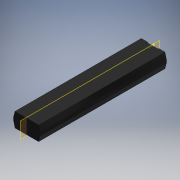
# Autodesk Inventor part: atmega_mold
Saved by Autodesk Inventor 2018 (Build 220112000, 112)
## iProperties
Created: 2017-04-13
Part Number: atmega_mold
Material: Generic
Document SubType Name: Modeling
Designer: kampe_000
Density: 1 g/cm^3
Appearance: Default
atmegaPinDistance: 2,540 mm
AtmegaChamfer_D2: 1,500 mm
AtmegaChamfer_D1: 0,400 mm
Author: kampe_000
Autodesk Inventor part; units mm, degrees
ref_plane "YZ Plane" through (0, 0, 0) normal (1, 0, 0) x (0, 1, 0)
ref_plane "XZ Plane" through (0, 0, 0) normal (0, 1, 0) x (-1, 0, 0)
ref_plane "XY Plane" through (0, 0, 0) normal (0, 0, 1) x (1, 0, 0)
sketch "Sketch1" plane through (0, 0, 0) normal (0, 1, 0) x (-1, 0, 0)
  line L0 (0, 0) -> (7.3, 0)
  line L1 (7.3, 0) -> (7.3, -34.6)
  line L2 (7.3, -34.6) -> (0, -34.6)
  line L3 (0, -34.6) -> (0, 0)
  dimension "d0" = 7.3
  dimension "d1" = 34.6
  constraints: 8 end point, 2 parallel, 1 horizontal, 1 perpendicular
  measures "d0" distance of L1.end L2.end
  measures "d1" distance of L0.end L1.end
extrude "Extrusion1" add sketch "Sketch1" along normal blind 4
chamfer "Chamfer1" distance 0.4 distance2 1.5 1 edges at (0, 4, -17.3) measured on face at (-0.5, 4, -17.3)
chamfer "Chamfer2" distance 0.4 distance2 1.5 1 edges at (0, 0, -17.3) measured on face at (-0.5, 0, -17.3)
chamfer "Chamfer3" distance 0.4 distance2 1.5 1 edges at (-7.3, 4, -17.3) measured on face at (-6.8, 4, -17.3)
chamfer "Chamfer4" distance 0.4 distance2 1.5 1 edges at (-7.3, 0, -17.3) measured on face at (-6.8, 0, -17.3)
ref_plane "Work Plane1" through (-3.65, 2.5, 0) normal (1, 0, 0) x (0, 0, -1)
hole "Hole1" at (-3.65, 4, -34.6) direction (0, -1, 0) diameter 3 depth 0.2
sketch "Sketch3" plane through (0, 2.5, 0) normal (1, 0, 0) x (0, 0, -1)
  line L0 (34.6, -1) -> (34.6, 0) projected
  line L1 (34.6, -0.5) -> (0, -0.5) construction
  line L2 (0, -1) -> (0, 0) projected
  line L3 (2.73, -0.375) -> (3.93, -0.375)
  line L4 (3.93, -0.375) -> (3.93, -0.625)
  line L5 (3.93, -0.625) -> (2.73, -0.625)
  line L6 (2.73, -0.625) -> (2.73, -0.375)
  line L7 (2.73, -0.375) -> (3.93, -0.625) construction
  line L8 (3.93, -0.375) -> (2.73, -0.625) construction
  point P0 (0, -2.5)
  point P1 (17.3, -0.5)
  point P2 (3.33, -0.5)
  dimension "d30" = 13.97
  dimension "d31" = 1.2
  dimension "d32" = 0.25
  constraints: 14 end point, 5 midpoint, 2 parallel, 1 horizontal, 1 perpendicular, 1 point on line
  measures "d30" distance of point (17.3, -0.5) point (3.33, -0.5)
  measures "d31" distance of L3.start L3.end
  measures "d32" distance of L3.end L4.end
extrude "Extrusion2" cut sketch "Sketch3" against normal through all
pattern_linear "Rectangular Pattern1" count 12 spacing 2.54 along (0, 0, -1) of "Extrusion2"
equation "\"d4\" = AtmegaChamfer_D1"
equation "\"d5\" = AtmegaChamfer_D2"
equation "\"d7\" = AtmegaChamfer_D1"
equation "\"d8\" = AtmegaChamfer_D2"
equation "\"d10\" = AtmegaChamfer_D1"
equation "\"d11\" = AtmegaChamfer_D2"
equation "\"d13\" = AtmegaChamfer_D1"
equation "\"d14\" = AtmegaChamfer_D2"
equation "\"d30\" = 0.5 * Atmega28PinsDistance - atmegaPinSpacing"
equation "\"d31\" = atmegaPinWidth1"
equation "\"d37\" = atmegaPinSpacing"
equation "\"AtmegaChamfer_D1\" = 0.4"
equation "\"atmegaPinDistance\" = 2.54"
equation "\"Thickness\" = 0.25"
equation "\"BendRadius\" = 0.25"
equation "\"BendReliefWidth\" = 0.25"
equation "\"BendReliefDepth\" = 0.125"
equation "\"CornerReliefSize\" = 1"
equation "\"MinimumRemnant\" = 0.5"
equation "\"TransitionRadius\" = 0.25"
equation "\"JacobiRadiusSize\" = 0.25"
equation "\"GapSize\" = 0.25"
equation "\"atmegaPinThickness\" = 0.3"
equation "\"atmegaPinWidth1\" = 1.2"
equation "\"atmegaPinWidth2\" = 0.5"
equation "\"atmegaEndPinWidth\" = 0.9"
equation "\"atmegaPinBendAngle\" = 80deg"
equation "\"atmegaPinBaseWidth\" = 8"
equation "\"atmegaSeatingPlaneDistance\" = 3.2"
equation "\"d27\" = atmegaPinBaseWidth"
equation "\"d28\" = atmegaPinWidth1"
equation "\"d29\" = 0.25"
equation "\"d40\" = BendReliefWidth"
equation "\"d41\" = BendReliefDepth"
equation "\"d42\" = MinimumRemnant"
equation "\"d43\" = TransitionRadius"
equation "\"d45\" = 90deg"
equation "\"d46\" = BendRadius"
equation "\"d47\" = CornerReliefSize"
equation "\"d48\" = GapSize"
equation "\"d49\" = JacobiRadiusSize"
equation "\"d50\" = Thickness"
equation "\"d51\" = 0"
equation "\"d52\" = atmegaSeatingPlaneDistance"
equation "\"d54\" = 0.5 * atmegaPinWidth2"
equation "\"d56\" = 2.5"
equation "\"d44\" = atmegaPinLenght"
equation "\"Atmega28PinsDistance\" = 13 * atmegaPinSpacing"
equation "\"atmegaPinSpacing\" = 2.54"
equation "\"AtmegaChamfer_D2\" = 1.5"
equation "\"atmegaPinLenght\" = 5.7"
body "Solid1"
